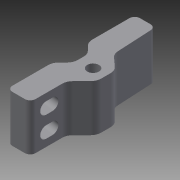
# Autodesk Inventor part: ExtruderSatoerCamArm
Saved by Autodesk Inventor 2015 SP1 (Build 190203100, 203)
## iProperties
Created: 2015-05-02
Part Number: ExtruderSatoerCamArm
Material: Generic
Document SubType Name: Modeling
Designer: Jack
Density: 1 g/cm^3
Appearance: Default
Author: Jack
Autodesk Inventor part; units mm, degrees
ref_plane "YZ Plane" through (0, 0, 0) normal (1, 0, 0) x (0, 1, 0)
ref_plane "XZ Plane" through (0, 0, 0) normal (0, 1, 0) x (-1, 0, 0)
ref_plane "XY Plane" through (0, 0, 0) normal (0, 0, 1) x (1, 0, 0)
sketch "Sketch1" plane through (0, 0, 0) normal (0, 0, 1) x (1, 0, 0)
  line L0 (-0.0471, -0.0824) -> (104.8002, -0.0824) construction
  line L1 (104.8002, -0.0824) -> (104.8002, -53.0533) construction
  line L2 (104.8002, -53.0533) -> (-0.0471, -53.0533) construction
  line L3 (-0.0471, -53.0533) -> (-0.0471, -0.0824) construction
  line L4 (48.7, -18.9324) -> (48.7, -0.9324)
  line L5 (56.7, -0.9324) -> (57.6, -17.9324)
  line L6 (57.6, -36.0324) -> (57.6, -50.0324)
  line L7 (48.7, -50.0324) -> (57.6, -50.0324)
  line L8 (56.7, -0.9324) -> (48.7, -0.9324)
  line L9 (48.7, -18.9324) -> (52.7, -22.9324)
  line L10 (52.7, -22.9324) -> (52.7, -28.5324)
  line L11 (52.7, -28.5324) -> (48.7, -32.5324)
  line L12 (57.6, -36.0324) -> (63.4, -30.2324)
  line L13 (63.4, -30.2324) -> (63.4, -23.1492)
  line L14 (63.4, -23.1492) -> (57.6, -17.9324)
  line L15 (48.7, -32.5324) -> (48.7, -50.0324)
  point P0 (0, 0)
  dimension "d19" = 49.1
  dimension "d44" = 8
  dimension "d68" = 48.7
  dimension "d74" = 135
  dimension "d77" = 135
  dimension "d82" = 0.9
  dimension "d85" = 10.7
  dimension "d86" = 135
  dimension "d87" = 135
  dimension "d96" = 0.85
  dimension "d104" = 18
  dimension "d105" = 17.5
  dimension "d117" = 8.9
  dimension "d120" = 14
  dimension "d121" = 17
  dimension "d124" = 4
  constraints: 26 end point, 5 vertical, 2 horizontal, 1 horizontal alignment, 1 vertical alignment, 4 other
  measures "d19" distance between parallel lines of L8 L7
  measures "d44" distance of L5.start L4.end
  measures "d68" horizontal distance of point (0, 0) L4.end
  measures "d74" angle of L10 L9
  measures "d77" angle of L10 L11
  measures "d82" horizontal distance of L5.start L5.end
  measures "d85" distance between parallel lines of L10 L13
  measures "d86" angle of L5 L14
  measures "d87" angle of L6 L12
  measures "d96" vertical distance of L0.start L4.end
  measures "d104" distance of L4.start L4.end
  measures "d105" distance of L7.start L11.end
  measures "d117" distance of L7.start L6.end
  measures "d120" distance of L6.start L6.end
  measures "d121" vertical distance of L5.start L5.end
  measures "d124" distance between parallel lines of L4 L10
extrude "Extrusion2" add sketch "Sketch1" along normal blind 18
fillet "Fillet3" radius 2 4 edges at (56.7, -0.9324, 9) (48.7, -0.9324, 9) (57.6, -50.0324, 9) (48.7, -50.0324, 9)
fillet "Fillet4" radius 4 8 edges at (48.7, -18.9324, 9) (57.6, -17.9324, 9) (52.7, -22.9324, 9) (52.7, -28.5324, 9) (48.7, -32.5324, 9) (57.6, -36.0324, 9) (63.4, -30.2324, 9) (63.4, -23.1492, 9)
sketch "Sketch2" plane through (48.7, -48.0324, 0) normal (-1, 0, 0) x (0, 0, 1)
  line L0 (0, 0) -> (0, 13.8431) projected
  line L1 (18, 13.8431) -> (18, 0) projected
  line L2 (0, -2) -> (18, -2) projected
  line L3 (5, 1.1) -> (5, 7.9) construction
  line L4 (7.25, 1.1) -> (7.25, 7.9)
  line L5 (2.75, 7.9) -> (2.75, 1.1)
  arc A0 (2.75, 1.1) -> (7.25, 1.1) centre (5, 1.1) ccw
  arc A1 (7.25, 7.9) -> (2.75, 7.9) centre (5, 7.9) ccw
  line L6 (13, 7.9) -> (13, 1.1) construction
  line L7 (10.75, 7.9) -> (10.75, 1.1)
  line L8 (15.25, 1.1) -> (15.25, 7.9)
  arc A2 (15.25, 7.9) -> (10.75, 7.9) centre (13, 7.9) ccw
  arc A3 (10.75, 1.1) -> (15.25, 1.1) centre (13, 1.1) ccw
  point P0 (0, 48.0324)
  point P1 (5, 4.5)
  point P2 (13, 4.5)
  dimension "d129" = 4.5
  dimension "d130" = 6.8
  dimension "d131" = 3.1
  dimension "d132" = 5
  dimension "d133" = 5
  constraints: 16 end point, 8 point on circle, 8 tangent, 4 centre point, 3 parallel, 2 midpoint, 2 vertical, 1 equal radius, 1 horizontal alignment
  measures "d129" diameter of A1
  measures "d130" distance of L3.start L3.end
  measures "d131" distance from line of L2 L3.start
  measures "d132" distance from line of L0 point (5, 4.5)
  measures "d133" distance from line of L1 point (13, 4.5)
sketch "Sketch3" plane through (57.6, -48.0324, 18) normal (1, 0, 0) x (0, 0, -1)
  line L0 (5, 7.9) -> (5, 1.1) construction
  line L1 (13, 1.1) -> (13, 7.9) construction
  line L2 (5, 4.1) -> (5, 6.6) construction
  line L3 (7.25, 4.1) -> (7.25, 6.6)
  line L4 (2.75, 6.6) -> (2.75, 4.1)
  arc A0 (2.75, 4.1) -> (7.25, 4.1) centre (5, 4.1) ccw
  arc A1 (7.25, 6.6) -> (2.75, 6.6) centre (5, 6.6) ccw
  line L5 (13, 4.1) -> (13, 6.6) construction
  line L6 (10.75, 4.1) -> (10.75, 6.6)
  line L7 (15.25, 6.6) -> (15.25, 4.1)
  arc A2 (10.75, 4.1) -> (15.25, 4.1) centre (13, 4.1) ccw
  arc A3 (15.25, 6.6) -> (10.75, 6.6) centre (13, 6.6) ccw
  line L8 (0, -2) -> (18, -2) projected
  point P0 (18, 48.0324)
  point P1 (5, 5.35)
  point P2 (13, 5.35)
  dimension "d134" = 2.5
  dimension "d135" = 4.5
  dimension "d136" = 6.1
  constraints: 16 end point, 8 point on circle, 8 tangent, 4 centre point, 4 point on line, 3 parallel, 2 midpoint, 1 equal radius, 1 horizontal alignment
  measures "d134" distance of L2.start L2.end
  measures "d135" diameter of A1
  measures "d136" distance from line of L8 L2.start
loft "Loft1" cut profiles "Sketch2", "Sketch3" contours A0 L5 A1 L4 / L6 A3 L7 A2
loft "Loft2" cut profiles "Sketch2", "Sketch3" contours A2 L8 A3 L7 / A0 L4 A1 L3
sketch "Sketch4" plane through (0, 0, 0) normal (0, 0, -1) x (-1, 0, 0)
  line L0 (-63.4, -24.9314) -> (-63.4, -28.5756) projected
  line L1 (-50.7, -0.9324) -> (-54.8031, -0.9324) projected
  point P0 (0, 0)
  point P1 (-58.4, -26.6324)
  dimension "d145" = 25.7
  dimension "d146" = 5
  measures "d145" distance from line of L1 point (-58.4, -26.632)
  measures "d146" distance from line of L0 point (-58.4, -26.632)
hole "Hole1" at (58.4, -26.6324, 0) direction (0, 0, 1) diameter 4.5 end through all
body "Solid2"
